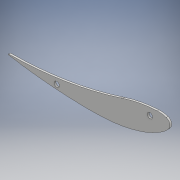
# Autodesk Inventor part: flap_m
Saved by Autodesk Inventor 2018.2 (Build 222227000, 227)
## iProperties
Created: 2018-03-11
Part Number: flap_m
Material: 一般
Document SubType Name: Modeling
Designer: ku_sk
Density: 1 g/cm^3
Appearance: 既定
Author: ku_sk
Autodesk Inventor part; units mm, degrees
ref_plane "YZ Plane" through (0, 0, 0) normal (1, 0, 0) x (0, 1, 0)
ref_plane "XZ Plane" through (0, 0, 0) normal (0, 1, 0) x (-1, 0, 0)
ref_plane "XY Plane" through (0, 0, 0) normal (0, 0, 1) x (1, 0, 0)
sketch "スケッチ1" plane through (0, 0, 0) normal (0, 1, 0) x (-1, 0, 0)
  arc A0 (348.9954, -50.1786) -> (348.3553, -42.2361) centre (348.3204, -46.2359) ccw projected
  arc A1 (182.359, -65.8653) -> (348.9954, -50.1786) centre (162.2533, 1040.6287) ccw projected
  arc A2 (135.1603, -65.3257) -> (182.359, -65.8653) centre (167.871, 731.467) ccw projected
  arc A3 (48.4731, -49.9165) -> (135.1603, -65.3257) centre (148.588, 261.756) ccw projected
  arc A4 (-1.5687, -25.3375) -> (48.4731, -49.9165) centre (107.173, 132.825) ccw projected
  arc A5 (-15.7749, -11.5429) -> (-1.5687, -25.3375) centre (31.9, 23.342) ccw projected
  arc A6 (-8.2474, 11.5993) -> (-15.7749, -11.5429) centre (-3.6695, -2.6851) ccw projected
  arc A7 (13.0537, 14.3873) -> (-8.2474, 11.5993) centre (10.0641, -45.5382) ccw projected
  arc A8 (91.047, 0) -> (13.0537, 14.3873) centre (-1.8944, -285.2401) ccw projected
  arc A9 (91.047, 0) -> (95.8009, -1.5381) centre (462.8125, 1140.9603) ccw projected
  arc A10 (95.8009, -1.5381) -> (348.3553, -42.2361) centre (355.7675, 807.7316) ccw projected
  point P0 (0, 0)
extrude "押し出し1" add sketch "スケッチ1" along normal mid plane 4
sketch "スケッチ2" plane through (0, -2, 0) normal (0, -1, 0) x (1, 0, 0)
  line L0 (0, 0) -> (-283.8627, -59.346)
  arc A0 (-348.9954, -50.1786) -> (-182.359, -65.8653) centre (-162.2533, 1040.6287) ccw projected
  circle A1 centre (-29.3651, -6.1392) radius 6
  circle A2 centre (-239.8151, -50.1371) radius 6
  dimension "d3" = 290
  dimension "d4" = 12
  dimension "d5" = 12
  dimension "d6" = 30
  dimension "d7" = 215
  constraints: 2 centre point, 2 end point, 2 point on line, 1 point on circle
  measures "d3" distance of L0.start L0.end
  measures "d4" diameter of A1
  measures "d5" diameter of A2
  measures "d6" distance of A1.centre L0.start
  measures "d7" distance of A1.centre A2.centre
extrude "押し出し2" cut sketch "スケッチ2" against normal through all
thicken "厚み1" operation cut thickness 3 both sides no extend neighbours no toward (0.1519877, 0, -0.9883824) faces at (-226.5779, 0.6667, -32.3934) (-92.1028, 0.6667, -0.3435) (-19.6698, -0.6667, 13.9839) (-3.4686, 0.6667, 14.0982) (9.3583, 0.6667, 11.1943) (14.4364, 0.6667, -13.3021) (-19.7763, 0.6667, -38.0608) (-76.8673, 0.6667, -57.648) (-177.1142, -0.6667, -65.9433) (-238.1449, 0.6667, -63.4427) (-351.8388, 0.6667, -48.1388)
